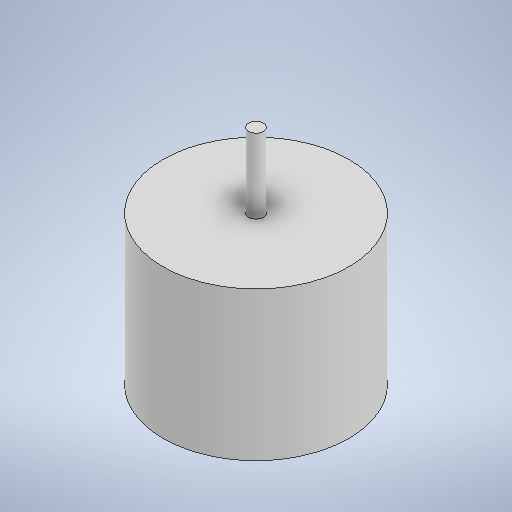
# Autodesk Inventor part: silnik
Saved by Autodesk Inventor 2025 (Build 290162000, 162)
## iProperties
Created: 2025-03-18
Part Number: silnik
Material: Generic
Document SubType Name: Modeling
Designer: HP
Density: 1 g/cm^3
Appearance: Default
Author: HP
Autodesk Inventor part; units mm, degrees
ref_plane "YZ Plane" through (0, 0, 0) normal (1, 0, 0) x (0, 1, 0)
ref_plane "XZ Plane" through (0, 0, 0) normal (0, 1, 0) x (-1, 0, 0)
ref_plane "XY Plane" through (0, 0, 0) normal (0, 0, 1) x (1, 0, 0)
sketch "Sketch5" plane through (0, 0, 0) normal (0, 1, 0) x (-1, 0, 0)
  circle A0 centre (0, 0) radius 12.5
  dimension "d14" = 25
  constraints: 1 centre point, 1 coincident
  measures "d14" diameter of A0
extrude "Extrusion3" add sketch "Sketch5" along normal blind 20
sketch "Sketch6" plane through (0, 20, 0) normal (0, 1, 0) x (1, 0, 0)
  circle A0 centre (0, 0) radius 1
  dimension "d18" = 2
  constraints: 1 centre point, 1 coincident
  measures "d18" diameter of A0
extrude "Extrusion4" add sketch "Sketch6" along normal blind 10
body "Solid3"
